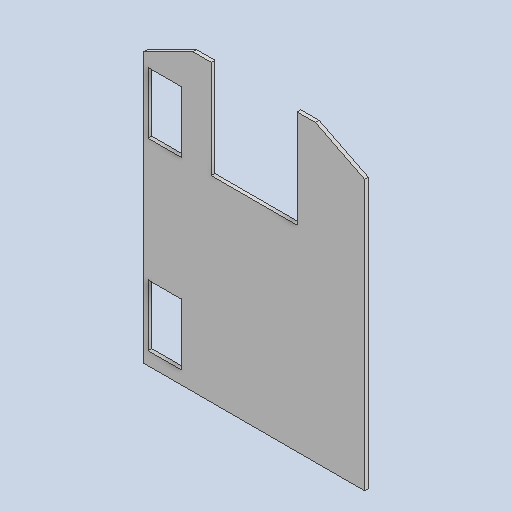
# Autodesk Inventor part: car platform
Saved by Autodesk Inventor 2023.2 (Build 272271030, 271C)
## iProperties
Created: 2023-06-19
Part Number: car platform
Material: Generic
Document SubType Name: Modeling
Designer: kao91
Density: 1 g/cm^3
Appearance: Default
Author: kao91
Autodesk Inventor part; units mm, degrees
ref_plane "YZ Plane" through (0, 0, 0) normal (1, 0, 0) x (0, 1, 0)
ref_plane "XZ Plane" through (0, 0, 0) normal (0, 1, 0) x (-1, 0, 0)
ref_plane "XY Plane" through (0, 0, 0) normal (0, 0, 1) x (1, 0, 0)
sketch "Sketch1" plane through (0, 0, 0) normal (0, 0, 1) x (1, 0, 0)
  line L0 (143.496, 22.8724) -> (143.496, -197.1276)
  line L1 (143.496, -197.1276) -> (-36.504, -197.1276)
  line L2 (-36.504, -197.1276) -> (-36.504, 22.8724)
  line L3 (144.25, -34) -> (144.25, 11) projected
  line L4 (113, 11) -> (113, -34) projected
  line L5 (144.25, -184) -> (144.25, -139) projected
  line L6 (113, -139) -> (113, -184) projected
  line L7 (-7, -143.5) -> (-7, -179.5) projected
  line L8 (-32, -179.5) -> (-32, -143.5) projected
  line L9 (-7, 6.5) -> (-7, -29.5) projected
  line L10 (-32, -29.5) -> (-32, 6.5) projected
  line L11 (145.25, -29.5) -> (145.25, 6.5)
  line L12 (112, 6.5) -> (112, -29.5)
  line L13 (112, -143.5) -> (112, -179.5)
  line L14 (-33, -179.5) -> (-33, -143.5)
  line L15 (-33, -29.5) -> (-33, 6.5)
  line L16 (-6, 6.5) -> (-6, -29.5)
  line L17 (-6, -143.5) -> (-6, -179.5)
  line L18 (145.25, -184) -> (145.25, -139)
  line L19 (145.25, -11.5) -> (112, -11.5)
  line L20 (115.125, 13.5) -> (142.125, 13.5)
  line L21 (142.125, 13.5) -> (142.125, -36.5)
  line L22 (142.125, -36.5) -> (115.125, -36.5)
  line L23 (115.125, -36.5) -> (115.125, 13.5)
  line L24 (115.125, 13.5) -> (142.125, -36.5) construction
  line L25 (142.125, 13.5) -> (115.125, -36.5) construction
  line L26 (145.25, -161.5) -> (112, -161.5)
  line L27 (115.125, -136.5) -> (142.125, -136.5)
  line L28 (142.125, -136.5) -> (142.125, -186.5)
  line L29 (142.125, -186.5) -> (115.125, -186.5)
  line L30 (115.125, -186.5) -> (115.125, -136.5)
  line L31 (115.125, -136.5) -> (142.125, -186.5) construction
  line L32 (142.125, -136.5) -> (115.125, -186.5) construction
  line L33 (-6, -161.5) -> (-33, -161.5)
  line L34 (-33, -136.5) -> (-6, -136.5)
  line L35 (-6, -136.5) -> (-6, -186.5)
  line L36 (-6, -186.5) -> (-33, -186.5)
  line L37 (-33, -186.5) -> (-33, -136.5)
  line L38 (-33, -136.5) -> (-6, -186.5) construction
  line L39 (-6, -136.5) -> (-33, -186.5) construction
  line L40 (-6, -11.5) -> (-33, -11.5)
  line L41 (-33, 13.5) -> (-6, 13.5)
  line L42 (-6, 13.5) -> (-6, -36.5)
  line L43 (-6, -36.5) -> (-33, -36.5)
  line L44 (-33, -36.5) -> (-33, 13.5)
  line L45 (-33, 13.5) -> (-6, -36.5) construction
  line L46 (-6, 13.5) -> (-33, -36.5) construction
  line L47 (143.496, 22.8724) -> (103.496, 42.8724)
  line L48 (3.496, 42.8724) -> (-36.504, 22.8724)
  line L49 (88.496, 42.8724) -> (88.496, -37.1276)
  line L50 (88.496, -37.1276) -> (18.496, -37.1276)
  line L51 (18.496, -37.1276) -> (18.496, 42.8724)
  line L52 (18.496, 122.8724) -> (88.496, -37.1276) construction
  line L53 (88.496, 122.8724) -> (18.496, -37.1276) construction
  line L54 (3.496, 42.8724) -> (18.496, 42.8724)
  line L55 (88.496, 42.8724) -> (103.496, 42.8724)
  point P0 (0, 0)
  point P1 (128.625, -11.5)
  point P2 (128.625, -161.5)
  point P3 (-19.5, -161.5)
  point P4 (-19.5, -11.5)
  point P5 (139, -143.5)
  point P6 (139, -179.5)
  point P7 (139, 6.5)
  point P8 (139, -29.5)
  dimension "d2" = 1
  dimension "d3" = 1
  dimension "d4" = 1
  dimension "d5" = 1
  dimension "d6" = 1
  dimension "d7" = 1
  dimension "d8" = 1
  dimension "d9" = 1
  dimension "d10" = 36
  dimension "d11" = 50
  dimension "d12" = 50
  dimension "d13" = 50
  dimension "d14" = 50
  dimension "d19" = 20
  dimension "d20" = 40
  dimension "d21" = 20
  dimension "d22" = 40
  dimension "d23" = 100
  dimension "d24" = 70
  dimension "d26" = 80
  dimension "d27" = 80
  dimension "d28" = 15
  dimension "d29" = 240
  constraints: 96 end point, 20 midpoint, 20 parallel, 6 horizontal, 6 perpendicular, 1 point on line
  measures "d2" distance between parallel lines of L3 L11
  measures "d3" distance between parallel lines of L4 L12
  measures "d4" distance between parallel lines of L6 L13
  measures "d5" distance between parallel lines of L8 L14
  measures "d6" distance between parallel lines of L10 L15
  measures "d7" distance between parallel lines of L9 L16
  measures "d8" distance between parallel lines of L7 L17
  measures "d9" distance between parallel lines of L5 L18
  measures "d10" distance of L11.start L11.end
  measures "d11" distance of L20.end L21.end
  measures "d12" distance of L27.end L28.end
  measures "d13" distance of L34.end L35.end
  measures "d14" distance of L41.end L42.end
  measures "d19" vertical distance of L47.end L0.start
  measures "d20" horizontal distance of L0.start L47.end
  measures "d21" vertical distance of L48.start L2.end
  measures "d22" horizontal distance of L48.start L2.end
  measures "d23" distance of L47.end L48.start
  measures "d24" distance of L49.end L50.end
  measures "d26" distance of L49.start L49.end
  measures "d27" distance of L50.end L51.end
  measures "d28" distance of L49.start L47.end
  measures "d29" vertical distance of L1.end L48.start
extrude "Extrusion1" add sketch "Sketch1" along normal blind 3 contours L0 L1 L2 L48 L54 L51 L50 L49 L55 L47 | L21 L22 L23 L19 | L19 L23 L20 L21 | L28 L29 L30 L26 | L26 L30 L27 L28
body "Solid1"
